Autodesk Inventor part; units mm, degrees
(part 2 of 2)
  spline S235 degree 2 poles (-17.5728, -19.2665) (-17.7787, -19.5007) (-17.965, -19.8714) (-17.9665, -20.0181) knots 0 0 0 1 2 2 2
  spline S236 degree 2 poles (-17.9665, -20.0181) (-17.9729, -20.1235) (-17.8946, -20.2869) (-17.8227, -20.3501) knots 0 0 0 1 2 2 2
  spline S237 degree 2 poles (-17.8227, -20.3501) (-17.7578, -20.4072) (-17.5924, -20.4622) (-17.4796, -20.4463) knots 0 0 0 1 2 2 2
  spline S238 degree 2 poles (-17.4796, -20.4463) (-17.382, -20.4335) (-17.1228, -20.279) (-17.0107, -20.1515) knots 0 0 0 1 2 2 2
  spline S239 degree 2 poles (-17.0107, -20.1515) (-16.8883, -20.0124) (-16.8032, -19.7707) (-16.8166, -19.6643) knots 0 0 0 1 2 2 2
  spline S240 degree 2 poles (-16.8166, -19.6643) (-16.8323, -19.556) (-16.9509, -19.3776) (-17.0483, -19.292) knots 0 0 0 1 2 2 2
  spline S241 degree 2 poles (-17.0483, -19.292) (-17.1294, -19.2206) (-17.3374, -19.1158) (-17.4111, -19.0921) knots 0 0 0 1 2 2 2
  spline S242 degree 2 poles (-17.4111, -19.0921) (-17.4295, -19.1129) (-17.5034, -19.1877) (-17.5728, -19.2665) knots 0 0 0 1 2 2 2
  dimension "d145" = 47.625
  constraints: 1 centre point, 1 coincident, 1 other
  measures "d145" diameter of A0
extrude "Text" cut sketch "Sketch26" against normal blind 2.54
split "Split1" plane through (0, 25.4, 0) removes the side toward (0, 1, 0)
equation "\"d103\" = hexDiameter"
equation "\"d110\" = centerLineForSpool"
equation "\"d111\" = centerLineForSpool"
equation "\"d112\" = holeForString"
equation "\"d121\" = centerLineForSpool"
equation "\"d122\" = holeForString"
equation "\"d125\" = knotHoleDiameter"
equation "\"d127\" = holeForString"
equation "\"d128\" = centerLineForSpool"
equation "\"d129\" = knotHoleDiameter"
equation "\"d130\" = knotHoleDepth"
equation "\"d86\" = spoolOverallHeight"
equation "\"d89\" = 0.5 * spoolOverallHeight"
equation "\"centerLineForSpool\" = 0.25 * spoolOverallHeight"
equation "\"holeForString\" = stringDiameter + clearanceForString"
equation "\"stringDiameter\" = 3.048"
equation "\"clearanceForString\" = 2.032"
equation "\"hexShaftDiameter\" = 12.7"
equation "\"clearanceForHexShaft\" = 0.508"
equation "\"hexDiameter\" = hexShaftDiameter + clearanceForHexShaft"
equation "\"spoolInteriorDiameter\" = 38.1"
equation "\"spoolInteriroRadius\" = 0.5 * spoolInteriorDiameter"
equation "\"spoolExteriorDiameter\" = 63.5"
equation "\"spoolExteriorRadius\" = 0.5 * spoolExteriorDiameter"
equation "\"hexHoleChamfer\" = 1.5875"
equation "\"stringHoleCenterFromHexShaft\" = 0.5 * hexDiameter + 0.5 * holeForString"
equation "\"textCircleDiameter\" = 0.75 * spoolExteriorDiameter"
equation "\"textHeight\" = 4.572"
equation "\"textDepth\" = 1.27"
equation "\"spoolOverallHeight\" = 50.8"
equation "\"d114\" = -spoolInteriroRadius"
equation "\"knotHoleDiameter\" = 9.525"
equation "\"d126\" = spoolInteriroRadius"
equation "\"metalWasherID\" = 26.67"
equation "\"metalWasherThickness\" = 0"
equation "\"spacerOD\" = 24.13"
equation "\"spacerThickness\" = 2.54"
equation "\"knotHoleDepth\" = 11.1125"
body "Solid3"
